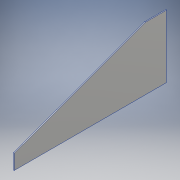
# Autodesk Inventor part: stay
Saved by Autodesk Inventor 2018.1 (Build 221171000, 171)
## iProperties
Created: 2017-10-18
Part Number: stay
Material: アルミニウム 6061
Document SubType Name: Modeling
Designer: kuwano
Density: 2.7 g/cm^3
Appearance: アルミニウム - フラット
Author: kuwano
Autodesk Inventor part; units mm, degrees
ref_plane "YZ Plane" through (0, 0, 0) normal (1, 0, 0) x (0, 1, 0)
ref_plane "XZ Plane" through (0, 0, 0) normal (0, 1, 0) x (-1, 0, 0)
ref_plane "XY Plane" through (0, 0, 0) normal (0, 0, 1) x (1, 0, 0)
sketch "スケッチ1" plane through (0, 0, 0) normal (1, 0, 0) x (0, 1, 0)
  line L0 (-55, 255) -> (-105, 255)
  line L1 (-105, 255) -> (-105, -255)
  line L2 (-105, -255) -> (105, -255)
  line L3 (105, -255) -> (105, -184.5964)
  line L4 (105, -184.5964) -> (-55, 255)
  line L5 (-147, 0) -> (147, 0) projected
  line L6 (0, -357) -> (0, 357) projected
  point P0 (0, 0)
  point P1 (-105, 0)
  point P2 (0, -255)
  dimension "d0" = 510
  dimension "d1" = 50
  dimension "d2" = 210
  dimension "d3" = 20
  constraints: 10 end point, 3 perpendicular, 2 midpoint, 2 point on line, 1 horizontal
  measures "d0" distance of L0.end L1.end
  measures "d1" distance of L0.start L0.end
  measures "d2" distance of L1.end L2.end
  measures "d3" angle of L1 L4
extrude "押し出し1" add sketch "スケッチ1" along normal blind 3
